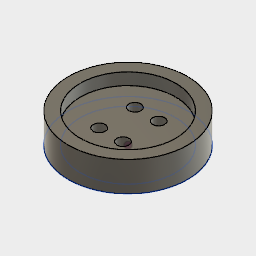
FPROJ_6 (Autodesk Fusion 360 design; units mm, degrees)
Autodesk Fusion 360 part; units mm, degrees
sketch "草图1" plane through (0, 0, 0) normal (0, 1, 0) x (1, 0, 0)
  circle A0 centre (0, 0) radius 10
  circle A1 centre (0, 0) radius 8
  dimension "d1" = 2
extrude "拉伸1" add sketch "草图1" along normal blind 3 contours A1 makes body 1
extrude "拉伸2" add sketch "草图1" along normal blind 5 separate body makes body 2
cylinder "圆柱体基本要素1" add diameter 2 height 20 placed x (1, 0, 0) y (0, 0, -1) z (0, 1, 0) at (20, 0, 1) separate body makes body 3
move_body "对齐1" bodies 3 to x (1, 0, 0) y (0, 1, 0) z (0, 0, 1) at (-20, 0, -1)
pattern_linear "R-阵列1" count 2 spacing 6 along (0, 0, 1) count 2 spacing 4 along (1, 0, 0) of bodies 3 makes body 4 at (0.995, 13.3333, 6.0996) makes body 5 at (4.995, 13.3333, 0.0996) makes body 6 at (4.995, 13.3333, 6.0996)
move_body "移动1" bodies 3 4 5 6 to x (1, 0, 0) y (0, 1, 0) z (0, 0, 1) at (-1.9322, 0, -3.0915)
combine "合并1" operation cut target body 1 tool bodies 3 4 5 6
combine "合并2" operation add target body 2 tool bodies 1
